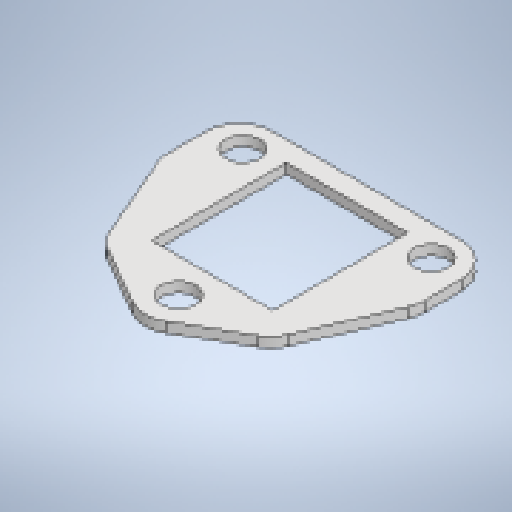
# Autodesk Inventor part: MNT-CDF-504 small tube flange
Saved by Autodesk Inventor 2025.1 (Build 291241020, 241B)
## iProperties
Created: 2025-01-13
Part Number: MNT-CDF-504 small tube flange
Material: Stainless Steel
Document SubType Name: Sheet Metal
Designer: user
Mass: 280.619 g
Surface Area: 364.406 cm^2
Volume: 35.0774 cm^3
Density: 8 g/cm^3
Sheet Metal Rule: AISI304 3mm Die 32
Sheet Metal Width: 0,000 mm
Sheet Metal Length: 0,000 mm
Sheet Metal Area: 0,000 mm^2
Appearance: Default
Author: user
Autodesk Inventor part; units mm, degrees
ref_plane "YZ Plane" through (0, 0, 0) normal (1, 0, 0) x (0, 1, 0)
ref_plane "XZ Plane" through (0, 0, 0) normal (0, 1, 0) x (-1, 0, 0)
ref_plane "XY Plane" through (0, 0, 0) normal (0, 0, 1) x (1, 0, 0)
sketch "Sketch6" plane through (0, 0, 0) normal (0, 0, 1) x (1, 0, 0)
  line L0 (18, 18) -> (-18, 18)
  line L1 (-18, 18) -> (-18, -18)
  line L2 (-18, -18) -> (18, -18)
  line L3 (18, -18) -> (18, 18)
  line L4 (18, 18) -> (-18, -18) construction
  circle A0 centre (0, -31) radius 5.05
  circle A1 centre (31, 14) radius 5.05
  circle A2 centre (-31, 14) radius 5.05
  line L5 (31, 14) -> (-31, 14) construction
  line L6 (-31, 14) -> (0, -31) construction
  line L7 (0, -31) -> (31, 14) construction
  line L8 (0, 18) -> (0, -18) construction
  line L9 (-41, 24) -> (41, 24)
  line L10 (41, 24) -> (41, 1)
  line L11 (41, 1) -> (25.1414, -25)
  line L12 (25.1414, -25) -> (0, -43.3896)
  line L13 (-41, 24) -> (-41, 1)
  line L14 (-41, 1) -> (-25.1414, -25)
  line L15 (-25.1414, -25) -> (0, -43.3896)
  point P0 (0, 0)
  point P1 (0, 0)
  point P2 (60, 0)
  dimension "d30" = 36
  dimension "d31" = 36
  dimension "d33" = 10.1
  dimension "d37" = 54.6443
  dimension "d43" = 13
  dimension "d44" = 13
  dimension "d45" = 6
  dimension "d46" = 10
  dimension "d47" = 10
  dimension "d48" = 10
  dimension "d49" = 23
  dimension "d50" = 7
  dimension "d51" = 10
  measures "d30" distance of L2.end L1.end
  measures "d31" distance of L1.end L1.start
  measures "d33" diameter of A0
  measures "d37" distance of L6.start L6.end
  measures "d43" distance from line of L2 L6.end
  measures "d44" distance from line of L1 L6.start
  measures "d45" distance between parallel lines of L0 L9
  measures "d46" distance from line of L13 L6.start
  measures "d47" distance from line of L6.end L15
  measures "d48" distance of L1.end L14.end
  measures "d49" distance of L9.start L13.end
  measures "d50" distance from line of L14.end L2
  measures "d51" distance between parallel lines of L5 L9
extrude "Plate3" add sketch "Sketch6" along normal blind 3
fillet "Corner Round1" radius 10 7 edges at (-41, 24, 1.5) (41, 24, 1.5) (41, 1, 1.5) (25.1414, -25, 1.5) (0, -43.3896, 1.5) (-25.1414, -25, 1.5) (-41, 1, 1.5)
equation "\"d41\" = Thickness"
equation "\"BendReliefWidth\" = Thickness"
equation "\"BendReliefDepth\" = 0.5 * Thickness"
equation "\"CornerReliefSize\" = 4 * Thickness"
equation "\"MinimumRemnant\" = 2 * Thickness"
equation "\"TransitionRadius\" = BendRadius"
equation "\"JacobiRadiusSize\" = BendRadius"
equation "\"GapSize\" = Thickness"
equation "\"Thickness\" = 3"
equation "\"BendRadius\" = 5"
body "Solid2"
